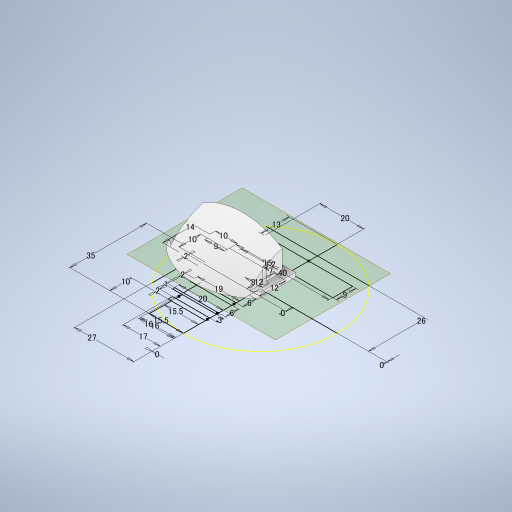
# Autodesk Inventor part: body back for main 2
Saved by Autodesk Inventor 2023 (Build 270158000, 158)
## iProperties
Created: 2022-10-08
Part Number: body back for main 2
Material: ABS プラスチック
Document SubType Name: Modeling
Designer: ellie
Density: 1.06 g/cm^3
Appearance: 積雪
Author: ellie
Autodesk Inventor part; units mm, degrees
ref_plane "YZ Plane" through (0, 0, 0) normal (1, 0, 0) x (0, 1, 0)
ref_plane "XZ Plane" through (0, 0, 0) normal (0, 1, 0) x (-1, 0, 0)
ref_plane "XY Plane" through (0, 0, 0) normal (0, 0, 1) x (1, 0, 0)
sketch "スケッチ1" plane through (0, 0, 0) normal (0, 1, 0) x (-1, 0, 0)
  circle A0 centre (0, 0) radius 35
  line L0 (0, 0) -> (0, -35)
  line L1 (0, 0) -> (0, 35)
  dimension "d0" = 70
  constraints: 4 end point, 2 point on circle, 2 vertical, 1 centre point, 1 coincident
  measures "d0" diameter of A0
revolve "回転1" add sketch "スケッチ1" angle 180 about axis through (0, 0, 0) along (0, 0, 1) picked at (-2.5961, -23.0408) contours L1 L0 A0
sketch "スケッチ5" plane through (0, 0, 0) normal (0, -1, 0) x (1, 0, 0)
  line L0 (-20, -22) -> (20, -22)
  line L1 (20, -22) -> (20, -13)
  line L2 (20, -13) -> (-20, -13)
  line L3 (-20, -13) -> (-20, -22)
  line L4 (-20, -15) -> (-20, -13)
  line L5 (0, 25) -> (-17, 25)
  line L6 (-17, 25) -> (-17, 23)
  line L7 (-17, 23) -> (0, 23)
  line L8 (0, 23) -> (0, 25)
  line L9 (0, 20) -> (-20, 20)
  line L10 (-20, 20) -> (-20, 19)
  line L11 (-20, 19) -> (0, 19)
  line L12 (0, 19) -> (0, 20)
  line L13 (0, 13) -> (-19, 13)
  line L14 (-19, 13) -> (-19, 11)
  line L15 (-19, 11) -> (0, 11)
  line L16 (0, 11) -> (0, 13)
  line L17 (0, 5) -> (-23, 5)
  line L18 (-23, 5) -> (-23, 3)
  line L19 (-23, 3) -> (0, 3)
  line L20 (0, 3) -> (0, 5)
  circle A0 centre (0, 0) radius 35 projected
  circle A1 centre (0, 0) radius 35 projected
  line L21 (0, 35) -> (0, -35)
  line L22 (35, 0) -> (-35, 0)
  line L23 (-32, 2) -> (-23, 2)
  line L24 (-23, 2) -> (-23, -8)
  line L25 (-23, -8) -> (-32, -8)
  line L26 (-32, -8) -> (-32, 2)
  line L27 (-23, -8.0262) -> (-23, 2)
  line L28 (-27, 22.2711) -> (-27, -22.2711)
  line L29 (-15.5, 25) -> (0, 25)
  line L30 (0, 25) -> (0, 35)
  line L31 (0, 35) -> (-15.5, 35)
  line L32 (-15.5, 35) -> (-15.5, 25)
  line L33 (-15.5, 23) -> (0, 23)
  line L34 (0, 23) -> (0, 20)
  line L35 (0, 20) -> (-15.5, 20)
  line L36 (-15.5, 20) -> (-15.5, 23)
  line L37 (-16, 13) -> (0, 13)
  line L38 (0, 13) -> (0, 19)
  line L39 (0, 19) -> (-16, 19)
  line L40 (-16, 19) -> (-16, 13)
  line L41 (-16, 11) -> (0, 11)
  line L42 (0, 11) -> (0, 5)
  line L43 (0, 5) -> (-16, 5)
  line L44 (-16, 5) -> (-16, 11)
  line L45 (-23, -3) -> (-39.6865, -3)
  line L46 (-23, -3) -> (-7.8337, -3)
  line L47 (-8, 3) -> (-23, 3)
  line L48 (-23, 3) -> (-23, -9)
  line L49 (-23, -9) -> (-8, -9)
  line L50 (-8, -9) -> (-8, 3)
  line L51 (-8, 3) -> (-23, -9) construction
  line L52 (-23, 3) -> (-8, -9) construction
  line L53 (-23, 4) -> (-33, 4)
  line L54 (-33, 4) -> (-33, -10)
  line L55 (-33, -10) -> (-23, -10)
  line L56 (-23, -10) -> (-23, 4)
  line L57 (-23, 4) -> (-33, -10) construction
  line L58 (-33, 4) -> (-23, -10) construction
  line L59 (-8, 3) -> (-1, 3)
  line L60 (-1, 3) -> (-1, -9)
  line L61 (-1, -9) -> (-8, -9)
  line L62 (-8, -9) -> (-8, 3)
  line L63 (-8, 3) -> (-1, -9) construction
  line L64 (-1, 3) -> (-8, -9) construction
  line L65 (-23, 2) -> (-27, 2)
  line L66 (-23, -8) -> (-27, -8)
  line L67 (-23, 4) -> (-27, 4)
  line L68 (-23, -10) -> (-27, -10)
  line L69 (23.4307, -26) -> (-23.4307, -26)
  line L70 (-8, 3) -> (-6.8, 3)
  line L71 (-6.8, 3) -> (-6.8, -9)
  line L72 (-6.8, -9) -> (-8, -9)
  line L73 (-8, -9) -> (-8, 3)
  line L74 (-3, 5) -> (0, 5)
  line L75 (0, 20) -> (-4, 20)
  line L76 (-4, 19) -> (0, 19)
  line L77 (0, 19) -> (0, 20)
  line L78 (-6, 5) -> (-1, 5)
  line L79 (-1, 3) -> (-6, 3)
  point P0 (0, -22)
  point P1 (0, -13)
  point P2 (0, 24)
  point P3 (0, 19.5)
  point P4 (0, 12)
  point P5 (0, 4)
  point P6 (-20, -17.5)
  point P7 (-27, -0.5262)
  point P8 (-27, -8)
  point P9 (-15.5, 21.5)
  point P10 (-15.5, 31.3807)
  point P11 (0, 25)
  point P12 (0, 23)
  point P13 (0, 11)
  point P14 (0, 13)
  point P15 (-27, 0)
  point P16 (-32, 0)
  point P17 (-23, 0)
  point P18 (-15.5, -3)
  point P19 (-28, -3)
  point P20 (-4.5, -3)
  point P21 (-8, -9)
  point P22 (-8, 3)
  point P23 (-27, 0.5)
  point P24 (-28, 0.4738)
  point P25 (-28, -11.5262)
  point P26 (-27, -11.5)
  point P27 (-23, 2)
  point P28 (-23, 2)
  point P29 (-8, 0)
  point P30 (-1, 0)
  point P31 (0, 19)
  point P32 (0, 20)
  point P33 (-27, -10)
  point P34 (-27, 4)
  dimension "d12" = 40
  dimension "d13" = 9
  dimension "d23" = 17
  dimension "d24" = 2
  dimension "d27" = 20
  dimension "d28" = 1
  dimension "d30" = 19
  dimension "d31" = 2
  dimension "d33" = 2
  dimension "d88" = 0
  dimension "d89" = 0
  dimension "d90" = 13
  dimension "d92" = 20
  dimension "d93" = 10
  dimension "d97" = 9
  dimension "d98" = 10
  dimension "d113" = 27
  dimension "d122" = 15.5
  dimension "d123" = 35
  dimension "d124" = 3
  dimension "d125" = 15.5
  dimension "d126" = 6
  dimension "d127" = 6
  dimension "d128" = 16
  dimension "d129" = 16
  dimension "d147" = 12
  dimension "d149" = 8
  dimension "d151" = 15
  dimension "d161" = 14
  dimension "d162" = 10
  dimension "d164" = 12
  dimension "d165" = 7
  dimension "d170" = 26
  dimension "d175" = 1.2
  dimension "d207" = 0
  constraints: 158 end point, 31 parallel, 20 horizontal, 17 perpendicular, 16 point on line, 15 midpoint, 10 collinear, 1 vertical, 20 other
  measures "d12" distance of L2.end L1.end
  measures "d13" distance of L1.end L0.end
  measures "d23" distance of L7.end L6.end
  measures "d24" distance of L6.end L5.end
  measures "d27" distance of L11.end L10.end
  measures "d28" distance of L10.end L9.end
  measures "d30" distance of L15.end L14.end
  measures "d31" distance of L14.end L13.end
  measures "d33" distance of L18.end L17.end
  measures "d89" distance from line of point (0, 0) L22
  measures "d90" distance from line of L0 point (0, -35)
  measures "d92" distance of the line from the sketch origin of L3
  measures "d93" distance from line of L5 point (0, 35)
  measures "d97" distance of L24.end L25.end
  measures "d98" distance of L23.end L24.end
  measures "d113" distance of the line from the sketch origin of L28
  measures "d122" distance of the line from the sketch origin of L32
  measures "d123" distance between parallel lines of L31 L22
  measures "d124" distance of L33.end L34.end
  measures "d126" distance of L38.end L37.end
  measures "d127" distance of L41.end L42.end
  measures "d128" distance of the line from the sketch origin of L44
  measures "d129" distance of the line from the sketch origin of L40
  measures "d147" distance of L48.end L47.end
  measures "d149" distance of the line from the sketch origin of L50
  measures "d151" distance between parallel lines of L50 L24
  measures "d161" distance between parallel lines of L55 L53
  measures "d162" distance between parallel lines of L48 L54
  measures "d164" distance between parallel lines of L61 L59
  measures "d165" distance between parallel lines of L50 L60
  measures "d170" distance between parallel lines of L69 L22
  measures "d175" distance of L71.end L72.end
  measures "d207" distance between parallel lines of L47 L19
extrude "GNSボード" cut sketch "スケッチ5" against normal blind 16 contours L8 L7 L6 L5
extrude "GNSボード止めるよう" cut sketch "スケッチ5" against normal blind 15 contours L21 L5 L32 A0 | L21 L9 L36 L7
extrude "アルミ板１" cut sketch "スケッチ5" against normal blind 17.5 contours L11 L10 L9 L12
extrude "メイン基板" cut sketch "スケッチ5" against normal blind 17.5 contours L15 L14 L13 L16
extrude "メイン止めるよう" cut sketch "スケッチ5" against normal blind 16.5 contours L17 L44 L15 L21 | L13 L40 L11 L21
extrude "アルミ板２" cut sketch "スケッチ5" against normal blind 19.5 contours L19 L18 L17 L20
extrude "電池ボックス入れ" cut sketch "スケッチ5" against normal blind 15 contours L3 L2 L21 L0 | L21 L2 L1 L0
extrude "side ut" cut sketch "スケッチ5" against normal blind 100 contours A0 L45 L54 L55 L28 | A0 L22 L54 L45 | L55 L54 L45 L26 L25 L28 | A0 L28 L53 L54 L22 | L54 L22 L26 L45 | L25 L26 L45 L28 | L54 L53 L28 L23 L26 L22 | L26 L22 L28 L45 | L22 L26 L23 L28
extrude "motor case" add sketch "スケッチ5" against normal blind 7 contours L55 L54 L45 L26 L25 L28 | L28 L25 L27 L48 L56 L55 | L50 L46 L24 L22 | L22 L24 L48 L19 L50 | L54 L22 L26 L45 | L28 L45 L24 L25 | L25 L26 L45 L28 | L24 L45 L28 L22 | L22 L28 L23 L24 | L50 L49 L48 L27 L24 L46 | L54 L53 L28 L23 L26 L22 | L26 L22 L28 L45 | L53 L18 L48 L23 L28 | L22 L26 L23 L28
extrude "bottom cut" cut sketch "スケッチ5" against normal blind 90 contours L69 A0 L21 | L21 A0 L69
extrude "motor" cut sketch "スケッチ5" against normal blind 6 contours L60 L61 L71 L22 | L22 L71 L19 L60 | L71 L61 L50 L22 | L22 L50 L19 L71 | L50 L46 L24 L22 | L22 L24 L48 L19 L50 | L28 L45 L24 L25 | L25 L26 L45 L28 | L24 L45 L28 L22 | L22 L28 L23 L24 | L50 L49 L48 L27 L24 L46 | L26 L22 L28 L45 | L22 L26 L23 L28
extrude "motor block" add sketch "スケッチ5" against normal blind 10 contours L71 L61 L50 L22 | L22 L50 L19 L71
sketch "スケッチ27" plane through (-33, 0, -10) normal (-1, 0, 0) x (0, 0, 1)
  line L0 (14, 0) -> (0, 0) projected
  circle A0 centre (7, 0) radius 3
  point P0 (10, 0)
  dimension "d198" = 6
  constraints: 1 centre point, 1 midpoint
  measures "d198" diameter of A0
extrude "押し出し36" cut sketch "スケッチ27" against normal blind 27
mirror "ミラー13" about plane through (0, 0, 0) normal (1, 0, 0) of "メイン止めるよう", "メイン基板", "アルミ板１", "GNSボード止めるよう", "GNSボード", "アルミ板２", "motor", "motor case", "押し出し36", "電池ボックス入れ", "side ut"
ref_plane "作業平面5" through (-17, 17.5, 23) normal (0, -1, 0) x (1, 0, 0)
sketch "スケッチ29" plane through (-17, 17.5, 23) normal (0, -1, 0) x (1, 0, 0)
  line L0 (32.5, 2) -> (1.5, 2) projected
  line L1 (1.5, 0) -> (32.5, 0) projected
  line L2 (32.5, -3) -> (1.5, -3) projected
  line L3 (1, -4) -> (33, -4) projected
  line L4 (33, -10) -> (1, -10) projected
  line L5 (33, -10) -> (33, -4) projected
  line L6 (1, -4) -> (33, -4) projected
  line L7 (1, -10) -> (1, -4) projected
  line L8 (1, -12) -> (33, -12) projected
  line L9 (33, -18) -> (1, -18) projected
  line L10 (33, -18) -> (33, -12) projected
  line L11 (1, -12) -> (33, -12) projected
  line L12 (1, -18) -> (1, -12) projected
  line L13 (18, -20) -> (40, -20) projected
  line L14 (-6, -20) -> (17, -20) projected
  line L15 (17, -18) -> (-6, -18) projected
  line L16 (-16, -23) -> (-15, -23) projected
  line L17 (-15, -23) -> (-15, -21) projected
  line L18 (-15, -21) -> (-6, -21) projected
  line L19 (-6, -21) -> (-6, -18) projected
  line L20 (-6, -18) -> (1, -18) projected
  line L21 (1, -18) -> (1, -12) projected
  line L22 (1, -12) -> (-2, -12) projected
  line L23 (-2, -12) -> (-2, -10) projected
  line L24 (-2, -10) -> (1, -10) projected
  line L25 (1, -10) -> (1, -4) projected
  line L26 (1, -4) -> (-3, -4) projected
  line L27 (-3, -4) -> (-3, -3) projected
  line L28 (-3, -3) -> (1.5, -3) projected
  line L29 (1.5, -3) -> (1.5, 0) projected
  line L30 (1.5, 0) -> (0, 0) projected
  line L31 (0, 0) -> (0, 2) projected
  line L32 (0, 2) -> (1.5, 2) projected
  line L33 (1.5, 2) -> (1.5, 8.3807) projected
  arc A0 (1.5, 8.3807) -> (-10, -0.7289) centre (17, -23) ccw projected
  line L34 (-10, -0.7289) -> (-10, -19) projected
  line L35 (-10, -19) -> (-16, -19) projected
  line L36 (-16, -19) -> (-16, -23) projected
  line L37 (49, -23) -> (50, -23) projected
  line L38 (50, -19) -> (50, -23) projected
  line L39 (44, -19) -> (50, -19) projected
  line L40 (44, -19) -> (44, -0.7289) projected
  arc A1 (44, -0.7289) -> (32.5, 8.3807) centre (17, -23) ccw projected
  line L41 (32.5, 8.3807) -> (32.5, 2) projected
  line L42 (32.5, 2) -> (34, 2) projected
  line L43 (34, 2) -> (34, 0) projected
  line L44 (34, 0) -> (32.5, 0) projected
  line L45 (32.5, 0) -> (32.5, -3) projected
  line L46 (32.5, -3) -> (37, -3) projected
  line L47 (37, -3) -> (37, -4) projected
  line L48 (37, -4) -> (33, -4) projected
  line L49 (33, -4) -> (33, -10) projected
  line L50 (33, -10) -> (36, -10) projected
  line L51 (36, -10) -> (36, -12) projected
  line L52 (36, -12) -> (33, -12) projected
  line L53 (33, -12) -> (33, -18) projected
  line L54 (33, -18) -> (40, -18) projected
  line L55 (40, -18) -> (40, -21) projected
  line L56 (40, -21) -> (49, -21) projected
  line L57 (49, -21) -> (49, -23) projected
  line L58 (40, -18) -> (-6, -18) projected
  line L59 (-4, -18) -> (38, -18)
  line L60 (38, -18) -> (38, 8.3807)
  line L61 (38, 8.3807) -> (-4, 8.3807)
  line L62 (-4, 8.3807) -> (-4, -18)
  circle A2 centre (17, -23) radius 35
  point P0 (-10, -0.7289)
  point P1 (44, -0.7289)
  point P2 (-4, 5)
  point P3 (38, 5)
  point P4 (37, -3)
  point P5 (38, -18)
  point P6 (32.5, 8.3807)
  point P7 (32.5, 8.3807)
  point P8 (1.5, 8.3807)
  point P9 (1.5, 8.3807)
  dimension "d209" = 2
  dimension "d210" = 2
  dimension "d211" = 26.3807
  dimension "d212" = 70
  constraints: 8 end point, 2 parallel, 1 centre point, 1 coincident, 1 horizontal, 1 perpendicular, 2 other
  measures "d209" distance between parallel lines of L19 L62
  measures "d210" distance between parallel lines of L60 L55
  measures "d211" distance between parallel lines of L9 L61
  measures "d212" diameter of A2
extrude "押し出し38" cut sketch "スケッチ29" against normal blind 30 contours A1 L40 L39 L38 L37 L57 L56 L55 L54 L60 | L62 L15 L19 L18 L17 L16 L36 L35 L34 A0 | A2 L34 L35 L36 L16 L17 L18 L19 L15 L9 L54 L55 L56 L57 L37 L38 L39 L40
sketch "スケッチ30" plane through (-17, 17.5, 23) normal (0, -1, 0) x (1, 0, 0)
  circle A0 centre (17, -23) radius 50
  line L0 (17, 2) -> (0, 2) projected
  line L1 (0, 0) -> (17, 0) projected
  line L2 (-16, -23) -> (-15, -23) projected
  line L3 (-15, -23) -> (-15, -21) projected
  line L4 (-15, -21) -> (-6, -21) projected
  line L5 (-6, -21) -> (-6, -18) projected
  line L6 (-6, -18) -> (1, -18) projected
  line L7 (1, -18) -> (1, -12) projected
  line L8 (1, -12) -> (-2, -12) projected
  line L9 (-2, -12) -> (-2, -10) projected
  line L10 (-2, -10) -> (1, -10) projected
  line L11 (1, -10) -> (1, -4) projected
  line L12 (1, -4) -> (-3, -4) projected
  line L13 (-3, -4) -> (-3, -3) projected
  line L14 (-3, -3) -> (1.5, -3) projected
  line L15 (1.5, -3) -> (1.5, 0) projected
  line L16 (1.5, 0) -> (0, 0) projected
  line L17 (0, 0) -> (0, 2) projected
  line L18 (0, 2) -> (1.5, 2) projected
  line L19 (1.5, 2) -> (1.5, 8.3807) projected
  arc A1 (1.5, 8.3807) -> (-10, -0.7289) centre (17, -23) ccw projected
  line L20 (-10, -0.7289) -> (-10, -19) projected
  line L21 (-10, -19) -> (-16, -19) projected
  line L22 (-16, -19) -> (-16, -23) projected
  line L23 (-4, -18) -> (-4, -1.1425) projected
  dimension "d215" = 100
  dimension "d218" = 5
  constraints: 1 centre point, 1 coincident
  measures "d215" diameter of A0
  measures "d218" distance between parallel lines of L23 L7
extrude "押し出し39" cut sketch "スケッチ30" along normal blind 100 contours A0 | L0 L17 L1 L15 L14 L13 L12 L11 L10 L9 L8 L7 L6 L5 L4 L3 L2 L22 L21 L20 A1 L19
sketch "スケッチ33" plane through (21, 17.5, 21.8575) normal (1, 0, 0) x (0, 0, -1)
  line L0 (16.8575, 0) -> (0, 0) projected
  line L1 (16.8575, 0) -> (16.8575, 10.05) projected
  line L2 (0, 0) -> (16.8575, 0)
  line L3 (16.8575, 0) -> (16.8575, 2)
  line L4 (0, 2) -> (0, 0)
  line L5 (16.8575, 17.141) -> (16.8575, 10.05) projected
  line L6 (0, 0) -> (-8.4534, 0) projected
  arc A0 (16.8575, 17.141) -> (-8.4534, 0) centre (21.8575, -17.5) ccw
  line L7 (-7.9835, 0) -> (0, 0)
  line L8 (16.8575, 2) -> (16.8575, 17.141)
  line L9 (16.8575, 0) -> (-8.4534, 0)
  line L10 (-8.4534, 0) -> (-8.4534, 2)
  line L11 (-8.4534, 2) -> (16.8575, 2)
  line L12 (16.8575, 2) -> (16.8575, 0)
  point P0 (21.8575, -17.5)
  point P1 (-7.2071, 2)
  point P2 (16.8575, 2)
  dimension "d236" = 2
  constraints: 18 end point, 3 parallel, 3 perpendicular, 2 horizontal, 2 point on circle, 2 point on line, 1 centre point, 1 collinear
  measures "d236" distance of L9.end L10.end
extrude "押し出し42" cut sketch "スケッチ33" against normal blind 3 contours L11 A0 L5 L1
sketch "スケッチ34" plane through (21, 17.5, 5) normal (0, 0, -1) x (-1, 0, 0)
  line L0 (3, 12.0973) -> (3, 2) projected
  line L1 (3, 2) -> (42, 2)
  line L2 (42, 0) -> (42, 10.05) projected
  arc A0 (42, 10.05) -> (3, 12.0973) centre (21, -17.5) ccw projected
  arc A1 (42, 10.05) -> (3, 12.0973) centre (21, -17.5) ccw
  line L3 (3, 12.0973) -> (3, 2)
  line L4 (42, 10.05) -> (42, 2)
  point P0 (3, 0)
  constraints: 6 end point, 2 point on circle, 1 centre point, 1 collinear, 1 horizontal, 1 point on line, 1 vertical
extrude "押し出し43" cut sketch "スケッチ34" against normal blind 3
sketch "スケッチ35" plane through (-21, 17.5, 5) normal (-1, 0, 0) x (0, 0, 1)
  line L0 (0, 0) -> (16.8575, 0) projected
  line L1 (0, 0) -> (16.8575, 0)
  line L2 (16.8575, 0) -> (16.8575, 2)
  line L3 (0, 2) -> (0, 0)
  line L4 (25.3109, 0) -> (16.8575, 0) projected
  line L5 (3, 11.431) -> (3, 16.5735) projected
  arc A0 (25.3109, 0) -> (3, 16.5735) centre (-5, -17.5) ccw
  arc A1 (25.3109, 0) -> (3, 16.5735) centre (-5, -17.5) ccw projected
  line L6 (25.3109, 0) -> (16.8575, 0)
  line L7 (3, 16.5735) -> (3, 2)
  line L8 (0, 0) -> (40.4212, 0)
  line L9 (40.4212, 0) -> (40.4212, 2)
  line L10 (40.4212, 2) -> (0, 2)
  line L11 (0, 2) -> (0, 0)
  point P0 (19.3875, 0)
  point P1 (3, 12.0296)
  point P2 (24.0646, 2)
  constraints: 18 end point, 3 horizontal, 3 parallel, 2 perpendicular, 2 point on circle, 1 centre point, 1 concentric
extrude "押し出し44" cut sketch "スケッチ35" against normal blind 3 contours L10 L7 L5 A0
sketch "スケッチ36" plane through (0, 17.5, 0) normal (0, -1, 0) x (1, 0, 0)
  line L0 (-16, 19) -> (-16, 13) projected
  line L1 (-20, 19) -> (0, 19) projected
  line L2 (0, 13) -> (-19, 13) projected
  line L3 (-21, 8) -> (-21, 5) projected
  line L4 (-16, 19) -> (-21, 19)
  line L5 (-21, 19) -> (-21, 13)
  line L6 (-21, 13) -> (-16, 13)
  line L7 (-16, 13) -> (-16, 19)
  line L8 (-16, 19) -> (-21, 13)
  line L9 (-16, 13) -> (-21, 19)
  circle A0 centre (-18.5, 16) radius 1
  line L10 (-21, 8) -> (18, 8) projected
  line L11 (0, 35) -> (0, -35) projected
  point P0 (0, 0)
  point P1 (-21, 20.0935)
  point P2 (-18, 8)
  dimension "d232" = 2
  dimension "d233" = 8
  constraints: 12 end point, 2 midpoint, 2 parallel, 1 centre point, 1 horizontal, 1 perpendicular, 1 point on line
  measures "d232" diameter of A0
  measures "d233" distance from line of point (-18.5, 16) L10
extrude "押し出し45" cut sketch "スケッチ36" against normal blind 100 contours A0 L9 L8 | L8 L9 A0 | A0 L8 L9 | L8 A0 L9
mirror "ミラー14" about plane through (0, 0, 0) normal (1, 0, 0) of "押し出し45"
